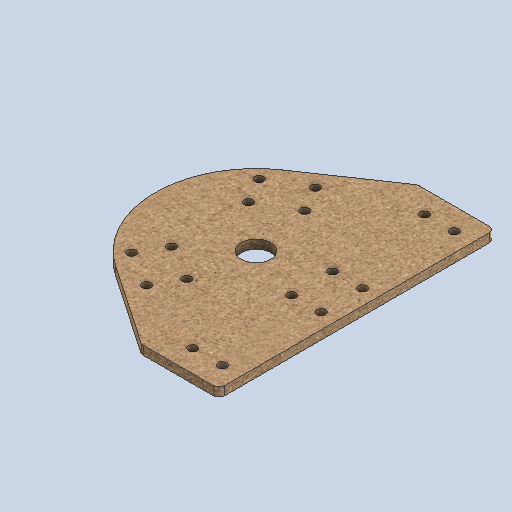
# Autodesk Inventor part: hand-grab-v1-MDF-air-Base
Saved by Autodesk Inventor 2025.1 (Build 291241000, 241)
## iProperties
Created: 2024-10-07
Part Number: hand-grab-v1-MDF-air-Base
Material: MDF 中密度繊維ボード
Document SubType Name: Modeling
Designer: haruy
Density: 0.8 g/cm^3
Appearance: ダンボール - 段ボール紙
Author: haruy
Autodesk Inventor part; units mm, degrees
ref_plane "YZ Plane" through (0, 0, 0) normal (1, 0, 0) x (0, 1, 0)
ref_plane "XZ Plane" through (0, 0, 0) normal (0, 1, 0) x (-1, 0, 0)
ref_plane "XY Plane" through (0, 0, 0) normal (0, 0, 1) x (1, 0, 0)
derived "hand-grab-v1-Sketch-Base.ipt"
sketch "スケッチ1" plane through (400, 0, 0) normal (1, 0, 0) x (0, 1, 0)
  circle A0 centre (0, 0) radius 120
  circle A1 centre (-109.5522, 63.25) radius 6.5
  line L0 (0, 0) -> (-109.5522, 63.25)
  line L1 (0, 0) -> (0, 120)
  line L2 (246.0862, 200) -> (-251.4603, 200)
  circle A2 centre (145, 60) radius 254.573
  circle A3 centre (-67.6203, 200) radius 6.5
  line L3 (0, 0) -> (-120, 0)
  line L4 (249, 9.15) -> (187, 9.15)
  line L5 (187, 9.15) -> (187, -9.15)
  line L6 (187, -9.15) -> (249, -9.15)
  line L7 (249, -9.15) -> (249, 9.15)
  line L8 (187, 5.15) -> (179, 5.15)
  line L9 (179, 5.15) -> (179, -4.85)
  line L10 (179, -4.85) -> (187, -4.85)
  line L11 (187, -4.85) -> (187, 5.15)
  line L12 (179, 3.15) -> (174, 3.15)
  line L13 (174, 3.15) -> (174, -2.85)
  line L14 (174, -2.85) -> (179, -2.85)
  line L15 (179, -2.85) -> (179, 3.15)
  line L16 (174, 2.65) -> (159, 2.65)
  line L17 (159, 2.65) -> (159, -2.35)
  line L18 (159, -2.35) -> (174, -2.35)
  line L19 (174, -2.35) -> (174, 2.65)
  line L20 (187, 34.15) -> (184, 34.15)
  line L21 (184, 34.15) -> (184, -43.5182)
  line L22 (184, -43.5182) -> (187, -43.5182)
  line L23 (187, -43.5182) -> (187, 34.15)
  circle A4 centre (150, 65) radius 4
  circle A5 centre (150, 65) radius 14
  line L24 (187, 34.15) -> (192, 34.15)
  line L25 (192, 34.15) -> (192, 14.15)
  line L26 (192, 14.15) -> (187, 14.15)
  line L27 (187, 14.15) -> (187, 34.15)
  line L28 (184, 34.15) -> (147.5804, 61.8148)
  line L29 (151.3533, 68.7641) -> (192, 54.15)
  line L30 (192, 54.15) -> (192, 34.15)
  line L31 (239.3868, 130) -> (-239.3868, 130)
  circle A6 centre (-109.5522, 63.25) radius 4
  circle A7 centre (150, 65) radius 9
  line L32 (-106.0881, 61.25) -> (-113.0163, 65.25)
  line L33 (170, 36) -> (155, 36)
  circle A8 centre (155, 36) radius 5
  circle A9 centre (155, 36) radius 9
  circle A10 centre (-90.698, 156.1969) radius 6.5
  circle A11 centre (170, 36) radius 5
  line L34 (150, 65) -> (170, 36)
  circle A12 centre (170, 36) radius 9
  circle A13 centre (150, 65) radius 44.2278
  line L35 (150, 65) -> (155, 36)
  line L36 (150, 65) -> (-109.5522, 63.25)
  line L37 (-90.698, 156.1969) -> (150, 65)
  line L38 (150, 65) -> (157.5146, 21.4152)
  circle A14 centre (150, 65) radius 35.2278
  circle A15 centre (155.9855, 30.2844) radius 9
  line L39 (168.0777, 21.2844) -> (136, 21.2844)
  line L40 (175, 3.15) -> (175, -2.85)
  point P0 (-60, 0)
sketch "スケッチ2" plane through (0, 400, 0) normal (0, 1, 0) x (-1, 0, 0)
  circle A0 centre (0, 0) radius 120
  line L0 (0, 0) -> (-331.4625, 0) construction
  line L1 (67.5, -116.9134) -> (-135, 0)
  circle A1 centre (0, 0) radius 5
  line L2 (0, 0) -> (67.5, 116.9134) construction
  line L3 (0, 0) -> (67.5, -116.9134) construction
  line L4 (0, 0) -> (-135, 0)
  line L5 (17.0359, 37.507) -> (12.0359, 28.8468) construction
  line L6 (12.0359, 28.8468) -> (15.5, 26.8468) construction
  line L7 (15.5, 26.8468) -> (20.5, 35.507) construction
  line L8 (20.5, 35.507) -> (17.0359, 37.507)
  line L9 (20.5, 35.507) -> (15.5, 26.8468) construction
  line L10 (15.5, 26.8468) -> (18.9641, 24.8468) construction
  line L11 (18.9641, 24.8468) -> (23.9641, 33.507) construction
  line L12 (23.9641, 33.507) -> (20.5, 35.507)
  line L13 (14.5359, 33.1769) -> (21.4641, 29.1769) construction
  circle A2 centre (0, 0) radius 2.65 construction
  line L14 (16.8194, 37.632) -> (10.3194, 26.3737) construction
  line L15 (10.3194, 26.3737) -> (5.9893, 28.8737) construction
  line L16 (5.9893, 28.8737) -> (12.4893, 40.132) construction
  line L17 (12.4893, 40.132) -> (16.8194, 37.632)
  line L18 (28.5107, 30.882) -> (24.1806, 33.382)
  line L19 (22.0107, 19.6237) -> (28.5107, 30.882) construction
  line L20 (24.1806, 33.382) -> (17.6806, 22.1237) construction
  line L21 (17.6806, 22.1237) -> (22.0107, 19.6237) construction
  circle A3 centre (0, 0) radius 28.3207 construction
  line L22 (-41, 9.25) -> (-41, 4.25)
  line L23 (-41, 4.25) -> (-28, 4.25) construction
  line L24 (-28, 9.25) -> (-41, 9.25) construction
  line L25 (-28, 4.25) -> (-28, 9.25)
  line L26 (-41, -4.25) -> (-28, -4.25) construction
  line L27 (-41, -9.25) -> (-41, -4.25)
  line L28 (-28, -9.25) -> (-41, -9.25) construction
  line L29 (-28, -4.25) -> (-28, -9.25)
  line L30 (12.4893, -40.132) -> (16.8194, -37.632)
  line L31 (16.8194, -37.632) -> (10.3194, -26.3737) construction
  line L32 (5.9893, -28.8737) -> (12.4893, -40.132) construction
  line L33 (10.3194, -26.3737) -> (5.9893, -28.8737) construction
  line L34 (24.1806, -33.382) -> (17.6806, -22.1237) construction
  line L35 (28.5107, -30.882) -> (24.1806, -33.382)
  line L36 (22.0107, -19.6237) -> (28.5107, -30.882) construction
  line L37 (17.6806, -22.1237) -> (22.0107, -19.6237) construction
  line L38 (5.9893, 28.8737) -> (5.373, 27.8064)
  line L39 (22.0107, 19.6237) -> (21.3945, 18.5564) construction
  line L40 (-28, 9.25) -> (-26.7675, 9.25)
  line L41 (-28, -9.25) -> (-26.7675, -9.25)
  line L42 (5.9893, -28.8737) -> (2.1934, -22.2991) construction
  line L43 (22.0107, -19.6237) -> (21.3945, -18.5564) construction
  line L44 (13.6109, 31.5748) -> (3.6109, 14.2543) construction
  line L45 (3.6109, 14.2543) -> (-1.5853, 17.2543) construction
  line L46 (-1.5853, 17.2543) -> (8.4147, 34.5748) construction
  line L47 (8.4147, 34.5748) -> (13.6109, 31.5748)
  circle A4 centre (3.5128, 20.0844) radius 1.5
  circle A5 centre (8.5128, 28.7446) radius 1.5
  circle A6 centre (20.6372, 21.7446) radius 1.5
  circle A7 centre (15.6372, 13.0844) radius 1.5
  circle A8 centre (-29.15, 7) radius 1.5
  circle A9 centre (-19.15, 7) radius 1.5
  circle A10 centre (-19.15, -7) radius 1.5
  circle A11 centre (-29.15, -7) radius 1.5
  circle A12 centre (8.5128, -28.7446) radius 1.5
  circle A13 centre (3.5128, -20.0844) radius 1.5
  circle A14 centre (15.6372, -13.0844) radius 1.5
  circle A15 centre (20.6372, -21.7446) radius 1.5
  line L48 (1.0128, 15.7543) -> (13.6109, 31.5748) construction
  circle A16 centre (0, 0) radius 34.3835
  line L49 (-8, 47) -> (-188, 47)
  line L50 (-188, 47) -> (-188, 32)
  line L51 (-188, 32) -> (-8, 32)
  line L52 (-8, 32) -> (-8, 47)
  circle A17 centre (-18, 39.5) radius 1.5
  circle A18 centre (-28, 39.5) radius 1.5
  line L53 (-34.3835, 47) -> (-34.3835, 0)
  line L54 (-8, 47) -> (19.3201, 28.4422)
  line L55 (-8, -47) -> (-188, -47)
  line L56 (-188, -32) -> (-8, -32)
  circle A19 centre (-18, -39.5) radius 1.5
  circle A20 centre (-28, -39.5) radius 1.5
  line L57 (-34.3835, -47) -> (-34.3835, 0)
  line L58 (-8, -47) -> (19.3201, -28.4422)
  point P0 (19.3201, -28.4422)
  dimension "d3" = 3
  dimension "d4" = 3
  dimension "d5" = 10
  dimension "d6" = 10
  dimension "d7" = 7.5
  dimension "d8" = 7.5
  measures "d3" diameter of A17
  measures "d4" diameter of A18
  measures "d5" distance from line of A17.centre L52
  measures "d6" distance of A18.centre A17.centre
  measures "d7" distance from line of A17.centre L49
  measures "d8" distance from line of L49 A18.centre
ref_plane "作業平面1" through (400, 0, 0) normal (1, 0, 0) x (0, 1, 0)
ref_plane "作業平面2" through (0, 400, 0) normal (0, 1, 0) x (-1, 0, 0)
extrude "押し出し1" add sketch "スケッチ2" along normal blind 3 contours L49 L52 A16 L51 L53 | L51 A16 L53 | L54 A16 L52 | L57 L56 A16 L58 L55 | A16 L51 L52 | A16 L56 L57 | A16 L52 L51
fillet "フィレット1" radius 2 4 edges at (34.3835, 401.5, 47) (8, 401.5, 47) (34.3835, 401.5, -47) (8, 401.5, -47)
sketch "スケッチ3" plane through (0, 403, 0) normal (0, 1, 0) x (1, 0, 0)
  arc A0 (8.615, 47) -> (7.4912, 46.6544) centre (8.615, 45) ccw projected
  line L0 (7.4912, 46.6544) -> (-19.3201, 28.4422) projected
  arc A1 (-19.3201, 28.4422) -> (-19.3201, -28.4422) centre (0, 0) ccw projected
  line L1 (-19.3201, -28.4422) -> (7.4912, -46.6544) projected
  arc A2 (7.4912, -46.6544) -> (8.615, -47) centre (8.615, -45) ccw projected
  line L2 (8.615, -47) -> (32.3835, -47) projected
  arc A3 (32.3835, -47) -> (34.3835, -45) centre (32.3835, -45) ccw projected
  line L3 (34.3835, -45) -> (34.3835, 45) projected
  arc A4 (34.3835, 45) -> (32.3835, 47) centre (32.3835, 45) ccw projected
  line L4 (32.3835, 47) -> (8.615, 47) projected
  circle A5 centre (0, 0) radius 5 projected
  circle A6 centre (-20.6372, 21.7446) radius 1.5 projected
  circle A7 centre (-15.6372, 13.0844) radius 1.5 projected
  circle A8 centre (-3.5128, 20.0844) radius 1.5 projected
  circle A9 centre (-8.5128, 28.7446) radius 1.5 projected
  circle A10 centre (29.15, 7) radius 1.5 projected
  circle A11 centre (19.15, 7) radius 1.5 projected
  circle A12 centre (19.15, -7) radius 1.5 projected
  circle A13 centre (29.15, -7) radius 1.5 projected
  circle A14 centre (-20.6372, -21.7446) radius 1.5 projected
  circle A15 centre (-15.6372, -13.0844) radius 1.5 projected
  circle A16 centre (-8.5128, -28.7446) radius 1.5 projected
  circle A17 centre (-3.5128, -20.0844) radius 1.5 projected
  circle A18 centre (28, -39.5) radius 1.5 projected
  circle A19 centre (18, -39.5) radius 1.5 projected
  circle A20 centre (28, 39.5) radius 1.5 projected
  circle A21 centre (18, 39.5) radius 1.5 projected
equation "\"d8\" = d7"
